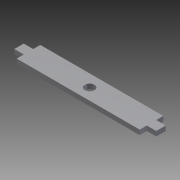
# Autodesk Inventor part: pieza lateral z refuerzo
Saved by Autodesk Inventor 2012 SP1 (Build 160190100, 190)
## iProperties
Created: 2014-12-27
Part Number: pieza lateral z refuerzo
Material: Default
Document SubType Name: Modeling
Designer: PRINCIPAL
Density: 1 g/cm^3
Author: PRINCIPAL
Autodesk Inventor part; units mm, degrees
ref_plane "YZ Plane" through (0, 0, 0) normal (1, 0, 0) x (0, 1, 0)
ref_plane "XZ Plane" through (0, 0, 0) normal (0, 1, 0) x (-1, 0, 0)
ref_plane "XY Plane" through (0, 0, 0) normal (0, 0, 1) x (1, 0, 0)
sketch "Boceto1" plane through (0, 0, 0) normal (0, 0, 1) x (1, 0, 0)
  line L0 (0, 0) -> (130, 0)
  line L1 (130, 0) -> (130, -25)
  line L2 (130, -25) -> (0, -25)
  line L3 (0, -25) -> (0, 0)
  dimension "d0" = 130
  dimension "d1" = 25
  constraints: 8 end point, 2 parallel, 1 horizontal, 1 perpendicular
  measures "d0" distance of L1.end L2.end
  measures "d1" distance of L0.end L1.end
extrude "Extrusión1" add sketch "Boceto1" along normal blind 5
sketch "Boceto2" plane through (0, 0, 5) normal (0, 0, 1) x (1, 0, 0)
  line L0 (130, 0) -> (130, -25) projected
  line L1 (0, -25) -> (0, 0) projected
  line L2 (-10, -7.5) -> (-10, -17.5)
  line L3 (140, -7.5) -> (140, -17.5)
  line L4 (0, -7.5) -> (0, -17.5)
  line L5 (130, -7.5) -> (130, -17.5)
  line L6 (140, -7.5) -> (130, -7.5)
  line L7 (0, -7.5) -> (-10, -7.5)
  line L8 (-10, -17.5) -> (0, -17.5)
  line L9 (130, -17.5) -> (140, -17.5)
  line L10 (0, 0) -> (130, 0) projected
  line L11 (130, -25) -> (0, -25) projected
  dimension "d5" = 10
  dimension "d6" = 10
  dimension "d12" = 7.5
  dimension "d13" = 10
  dimension "d14" = 10
  dimension "d15" = 7.5
  constraints: 16 end point, 5 parallel, 4 point on line, 2 horizontal
  measures "d5" distance between parallel lines of L0 L3
  measures "d6" distance between parallel lines of L1 L2
  measures "d12" distance between parallel lines of L10 L7
  measures "d13" distance between parallel lines of L7 L8
  measures "d14" distance between parallel lines of L6 L9
  measures "d15" distance between parallel lines of L11 L9
extrude "Extrusión2" add sketch "Boceto2" against normal blind 5 contours L6 L3 L9 L0 | L1 L8 L2 L7
sketch "Boceto3" plane through (0, 0, 5) normal (0, 0, 1) x (1, 0, 0)
  circle A0 centre (65, -12.8431) radius 5
  line L0 (130, -17.5) -> (130, -25) projected
  dimension "d9" = 10
  dimension "d16" = 65
  constraints: 1 centre point
  measures "d9" diameter of A0
  measures "d16" distance from line of L0 A0.centre
extrude "Extrusión3" cut sketch "Boceto3" against normal blind 5
